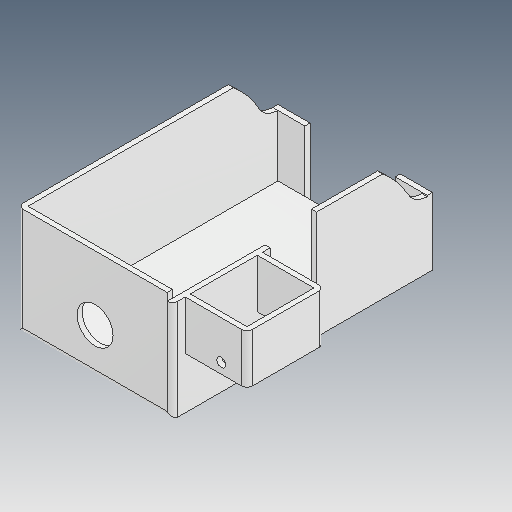
# Autodesk Inventor part: tension_sensor_cover
Saved by Autodesk Inventor 2025.2 (Build 292293000, 293)
## iProperties
Created: 2025-02-17
Part Number: tension_sensor_cover
Material: ABS Plastic
Document SubType Name: Modeling
Designer: email
Density: 1.06 g/cm^3
Appearance: Smooth - White
Author: email
Autodesk Inventor part; units mm, degrees
ref_plane "YZ Plane" through (0, 0, 0) normal (1, 0, 0) x (0, 1, 0)
ref_plane "XZ Plane" through (0, 0, 0) normal (0, 1, 0) x (-1, 0, 0)
sketch "Sketch1" plane through (0, 0, 0) normal (0, 1, 0) x (-1, 0, 0)
  line L0 (-60, -124) -> (0, -124)
  line L1 (0, -124) -> (0, 0)
  line L2 (-58, -33) -> (-58, -122)
  line L3 (-58, -122) -> (-40, -122)
  line L4 (-40, -122) -> (-40, -124)
  line L5 (-2, -2) -> (-2, -122)
  line L6 (-2, -122) -> (-20, -122)
  line L7 (-20, -122) -> (-20, -124)
  line L8 (-60, -35) -> (-60, -124)
  line L9 (-30, -124) -> (-30, 0) construction
  line L10 (-60, -124) -> (-60, 0)
  line L11 (-58, -124) -> (-58, -2)
  line L12 (-2, -2) -> (-58, -2)
  line L13 (-60, 0) -> (0, 0)
  line L14 (-84, -5) -> (-84, -35)
  line L15 (-84, -35) -> (-58, -35)
  line L16 (-58, -35) -> (-58, 0)
  line L17 (-82, -7) -> (-82, -33)
  line L18 (-82, -33) -> (-58, -33)
  line L19 (-58, -33) -> (-58, -2)
  line L20 (-82, -7) -> (-60, -7)
  line L21 (-84, -5) -> (-60, -5)
  point P0 (-57.4156, -121.9986)
  point P1 (-58, -122)
  point P2 (-60, -35)
  point P3 (-58, -38)
  point P4 (-58, -33)
  point P5 (-60, -33)
  point P6 (-60, -35)
  point P7 (-58, -33)
  point P8 (-58, -35)
  point P9 (-58, -35)
  dimension "d0" = 60
  dimension "d5" = 2
  dimension "d6" = 20
  dimension "d38" = 2
  dimension "d39" = 60
  dimension "d46" = 2
  dimension "d47" = 2
  dimension "d48" = 2
  dimension "d50" = 30
  dimension "d51" = 2
  dimension "d64" = 2
  dimension "d66" = 26
  constraints: 44 end point, 7 perpendicular, 6 point on line, 4 collinear, 3 parallel, 2 vertical, 1 horizontal, 1 midpoint
  measures "d0" distance of L1.end L10.end
  measures "d5" distance between parallel lines of L0 L6
  measures "d6" distance between parallel lines of L4 L7
  measures "d38" distance between parallel lines of L8 L2
  measures "d39" distance between parallel lines of L1 L8
  measures "d46" distance between parallel lines of L13 L12
  measures "d47" distance between parallel lines of L18 L15
  measures "d48" distance between parallel lines of L14 L17
  measures "d50" distance of L14.start L14.end
  measures "d51" distance between parallel lines of L21 L20
  measures "d64" distance between parallel lines of L1 L5
  measures "d66" distance of L14.end L15.end
extrude "Extrusion1" add sketch "Sketch1" against normal blind 2 contours L8 L15 L2 L11 L0 | L11 L3 L4 L0 | L10 L18 L2 L15 | L4 L3 L2 L11 L12 L5 L6 L7 L0 | L10 L13 L16 L11 L18 | L7 L6 L5 L12 L16 L13 L1 L0
extrude "Extrusion2" add sketch "Sketch1" along normal blind 40 contours L8 L15 L2 L11 L0 | L11 L3 L4 L0 | L10 L18 L2 L15 | L10 L13 L16 L11 L18 | L7 L6 L5 L12 L16 L13 L1 L0
sketch "Sketch2" plane through (0, -2, 0) normal (0, 0, 1) x (1, 0, 0)
  circle A0 centre (30, 17) radius 7
  line L0 (0, 42) -> (60, 42)
  line L1 (60, 0) -> (60, 42) projected
  point P0 (0, 2)
  point P1 (0, 42)
  point P2 (30, 42)
  dimension "d11" = 25
  dimension "d12" = 14
  dimension "d65" = 30
  constraints: 2 end point, 1 centre point, 1 midpoint, 1 vertical alignment
  measures "d11" distance from line of L0 A0.centre
  measures "d12" diameter of A0
  measures "d65" distance from line of L1 A0.centre
extrude "Extrusion3" cut sketch "Sketch2" against normal up to next
sketch "Sketch3" plane through (60, -2, 5.4121) normal (1, 0, 0) x (0, 0, -1)
  arc A0 (43.4121, 16) -> (61.4121, 16) centre (52.4121, 16) ccw
  line L0 (5.4121, 1.9762) -> (5.4121, 47)
  line L1 (61.4121, 16) -> (61.4121, 61)
  line L2 (61.4121, 61) -> (43.4121, 61)
  line L3 (43.4121, 61) -> (43.4121, 16)
  line L4 (5.4121, 47) -> (129.4107, 47) construction
  point P0 (5.4121, 2)
  point P1 (129.4107, 47)
  point P2 (5.4121, 0)
  dimension "d16" = 47
  dimension "d17" = 18
  dimension "d18" = 31
  dimension "d45" = 45
  constraints: 8 end point, 2 point on circle, 2 tangent, 2 vertical, 1 centre point, 1 parallel, 1 perpendicular, 1 point on line, 3 other
  measures "d16" distance from line of L0 A0.centre
  measures "d17" diameter of A0
  measures "d45" distance of L1.start L1.end
extrude "Extrusion4" cut sketch "Sketch3" against normal blind 2
ref_plane "Work Plane1" through (0, 18, 0) normal (0, -1, 0) x (1, 0, 0)
extrude "Extrusion7" add sketch "Sketch1" along normal up to surface (22 mm away) from surface at 18 contours L15 L14 L21 L10 L20 L17 L18
sketch "Sketch5" plane through (84, 18, -5) normal (1, 0, 0) x (0, 0, -1)
  line L0 (119, 22) -> (-5, 22) projected
  line L1 (33, 22) -> (33, -4) projected
  line L2 (-5, 22) -> (33, 22)
  line L3 (33, 22) -> (33, 19)
  line L4 (33, 19) -> (-5, 19)
  line L5 (-5, 19) -> (-5, 22)
  point P0 (-5, -18)
  dimension "d55" = 3
  constraints: 8 end point, 2 parallel, 1 horizontal, 1 perpendicular, 1 point on line
  measures "d55" distance between parallel lines of L0 L4
extrude "Extrusion8" cut sketch "Sketch5" against normal up to surface (26 mm away)
sketch "Sketch6" plane through (60, 18, -5) normal (0, 0, 1) x (1, 0, 0)
  circle A0 centre (14, 4) radius 1.75
  line L0 (24, 0) -> (24, 19) projected
  line L1 (0, 0) -> (24, 0) projected
  point P0 (-60, -18)
  dimension "d58" = 3.5
  dimension "d59" = 10
  dimension "d60" = 4
  constraints: 1 centre point
  measures "d58" diameter of A0
  measures "d59" distance from line of L0 A0.centre
  measures "d60" distance from line of L1 A0.centre
extrude "Extrusion9" cut sketch "Sketch6" against normal blind 10
fillet "Fillet1" radius 2 5 edges at (30, -2, 0) (0, 19, 0) (60, 17.5, 0) (84, 27.5, -35) (84, 27.5, -5)
sketch "Sketch7" plane through (0, 0, -122) normal (-1, 0, 0) x (0, 0, 1)
  line L0 (120, -2) -> (0, -2) projected
  line L1 (23, -2) -> (23, 23.6999)
  arc A0 (23, 23.6999) -> (30.364, 28.0218) centre (23, 32.1346) ccw
  arc A1 (67.8122, 50) -> (30.364, 28.0218) centre (67.8122, 7.1072) ccw
  line L2 (-2, 40) -> (120, 40) projected
  line L3 (-2, 50) -> (-2, 0) projected
  line L4 (67.8122, 50) -> (-2, 50)
  line L5 (-2, 50) -> (-2, -2)
  line L6 (-2, -2) -> (23, -2)
  point P0 (122, 0)
  point P1 (0, 50)
  point P2 (120, 40)
  point P3 (40.283, 40)
  point P4 (67.8122, 50)
  dimension "d67" = 25
  constraints: 8 end point, 4 point on circle, 2 centre point, 2 vertical, 1 collinear, 1 horizontal, 1 line through centre, 1 point on line, 1 tangent, 2 other
  measures "d67" distance between parallel lines of L3 L1
extrude "Extrusion10" cut sketch "Sketch7" against normal through all
sketch "Sketch8" plane through (0, 0, -99) normal (0, 0, -1) x (-1, 0, 0)
  line L0 (0, 23.6999) -> (0, -2) projected
  line L1 (0, -2) -> (-12.5, -2)
  line L2 (-12.5, -2) -> (-12.5, 23.6999)
  line L3 (-12.5, 23.6999) -> (0, 23.6999)
  line L4 (0, 23.6999) -> (0, -2)
  line L5 (-60, -2) -> (-60, 23.6999) projected
  line L6 (-60, -2) -> (-47.5, -2)
  line L7 (-47.5, -2) -> (-47.5, 24.1231)
  line L8 (-47.5, 24.1231) -> (-60, 24.1231)
  line L9 (-60, 24.1231) -> (-60, -2)
  point P0 (0, 0)
  point P1 (-60, 23.6999)
  dimension "d70" = 35
  constraints: 16 end point, 5 parallel, 2 horizontal, 2 perpendicular
  measures "d70" distance between parallel lines of L7 L2
extrude "Extrusion11" add sketch "Sketch8" along normal blind 2
body "Solid1"
